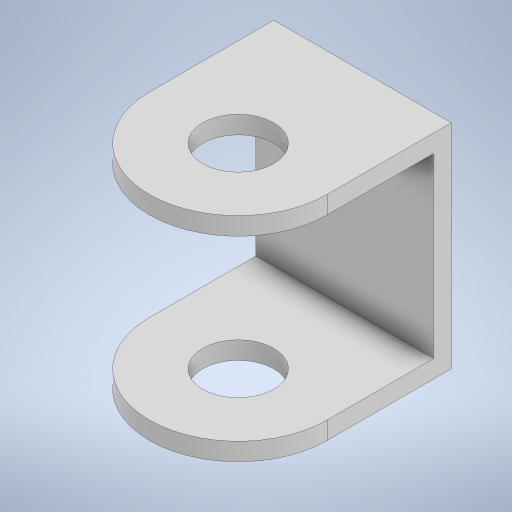
# Autodesk Inventor part: Langbektang houder
Saved by Autodesk Inventor 2023.2 (Build 272271000, 271)
## iProperties
Created: 2020-09-09
Part Number: Langbektang houder
Material: Generic
Document SubType Name: Modeling
Designer: nathan.bollaert
Density: 1 g/cm^3
Appearance: Default
Author: nathan.bollaert
Autodesk Inventor part; units mm, degrees
ref_plane "YZ Plane" through (0, 0, 0) normal (1, 0, 0) x (0, 1, 0)
ref_plane "XZ Plane" through (0, 0, 0) normal (0, 1, 0) x (-1, 0, 0)
ref_plane "XY Plane" through (0, 0, 0) normal (0, 0, 1) x (1, 0, 0)
sketch "Sketch1" plane through (0, 0, 0) normal (0, 1, 0) x (-1, 0, 0)
  line L0 (5, -5) -> (5, -12)
  line L1 (5, -12) -> (-5, -12)
  line L2 (-5, -12) -> (-5, -5)
  arc A0 (5, -5) -> (-5, -5) centre (0, -5) ccw
  circle A1 centre (0, -5) radius 2
  point P0 (0, 0)
  point P1 (0, 0)
  dimension "d230" = 10
  dimension "d231" = 7
  dimension "d232" = 5
  dimension "d234" = 4
  constraints: 6 end point, 3 coincident, 3 point on circle, 2 centre point, 1 horizontal, 1 parallel, 1 perpendicular
  measures "d230" distance of L0.end L1.end
  measures "d231" distance of L0.start L0.end
  measures "d232" radius of A0
  measures "d234" diameter of A1
extrude "Extrusion1" add sketch "Sketch1" along normal blind 1
sketch "Sketch2" plane through (0, 1, 0) normal (0, 1, 0) x (1, 0, 0)
  line L0 (5, 12) -> (-5, 12)
  line L1 (-5, 12) -> (-5, 11)
  line L2 (-5, 11) -> (5, 11)
  line L3 (5, 11) -> (5, 12)
  point P0 (0, 0)
  dimension "d237" = 1
  constraints: 8 end point, 2 coincident, 2 parallel, 1 horizontal, 1 perpendicular
  measures "d237" distance of L2.end L0.start
extrude "Extrusion2" add sketch "Sketch2" along normal blind 10
sketch "Sketch16" plane through (0, 11, 0) normal (0, 1, 0) x (1, 0, 0)
  line L0 (5, 5) -> (5, 12) projected
  line L1 (-5, 12) -> (-5, 5) projected
  line L2 (5, 12) -> (-5, 12)
  line L3 (-5, 12) -> (-5, 5)
  line L4 (5, 5) -> (5, 12)
  arc A0 (-5, 5) -> (5, 5) centre (0, 5) ccw
  circle A1 centre (0, 5) radius 2
  dimension "d244" = 4
  constraints: 6 end point, 2 centre point, 2 point on circle, 2 tangent, 1 coincident, 1 horizontal, 1 parallel, 1 perpendicular
  measures "d244" diameter of A1
extrude "Extrusion18" add sketch "Sketch16" along normal blind 1
body "Solid5"
